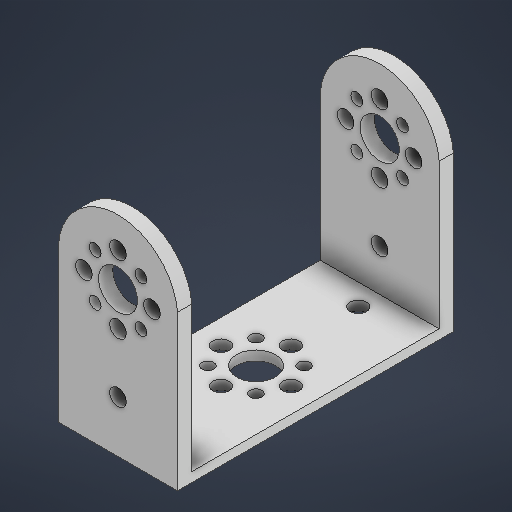
# Autodesk Inventor part: Medium FrameARRUMADO
Saved by Autodesk Inventor 2027 (Build 310192060, 192F)
## iProperties
Created: 2026-09-09
Part Number: Medium FrameARRUMADO
Material: Genérico
Document SubType Name: Modeling
Designer: joaop
Density: 1 g/cm^3
Appearance: Padrão
Author: joaop
Autodesk Inventor part; units mm, degrees
ref_plane "YZ Plane" through (0, 0, 0) normal (1, 0, 0) x (0, 1, 0)
ref_plane "XZ Plane" through (0, 0, 0) normal (0, 1, 0) x (-1, 0, 0)
ref_plane "XY Plane" through (0, 0, 0) normal (0, 0, 1) x (1, 0, 0)
sketch "Esboço1" plane through (0, 0, 0) normal (1, 0, 0) x (0, 1, 0)
  line L0 (0, 0) -> (50, 0)
  line L1 (50, 0) -> (50, 3)
  line L2 (50, 3) -> (2, 3)
  line L3 (2, 3) -> (2, 55)
  line L4 (2, 55) -> (50, 55)
  line L5 (50, 55) -> (50, 58)
  line L6 (50, 58) -> (0, 58)
  line L7 (0, 58) -> (0, 0)
  line L8 (2, 3) -> (0, 3)
  dimension "d84" = 52
  dimension "d85" = 3
  dimension "d86" = 3
  dimension "d87" = 3
  dimension "d90" = 2
  constraints: 18 end point, 3 point on line, 1 perpendicular
  measures "d84" distance between parallel lines of L2 L4
  measures "d85" distance of L4.end L5.end
  measures "d86" distance of L0.end L1.end
  measures "d87" distance from line of L2 L0.start
  measures "d90" distance between parallel lines of L7 L3
extrude "Extrusão1" add sketch "Esboço1" along normal blind 25
sketch "Esboço2" plane through (0, 0, 58) normal (0, 0, 1) x (1, 0, 0)
  line L0 (0, 0) -> (25, 0) projected
  circle A0 centre (12.5, 10.8) radius 1.75
  circle A1 centre (12.5, 30.4) radius 4.1
  circle A2 centre (12.5, 23.25) radius 1.75
  line L1 (12.5, 30.4) -> (16.5, 30.4) construction
  line L2 (12.5, 30.4) -> (19.3, 30.4) construction
  circle A3 centre (7.6917, 25.5917) radius 1.25
  circle A4 centre (19.65, 30.4) radius 1.75
  circle A5 centre (12.5, 37.55) radius 1.75
  circle A6 centre (5.35, 30.4) radius 1.75
  circle A7 centre (17.3083, 25.5917) radius 1.25
  circle A8 centre (17.3083, 35.2083) radius 1.25
  circle A9 centre (7.6917, 35.2083) radius 1.25
  line L3 (0, 0) -> (25, 0) projected
  line L4 (29.4538, 30.4) -> (-4.4538, 30.4)
  line L5 (12.5, 39.3) -> (12.5, 0)
  line L6 (12.5, 39.3) -> (12.5, 44)
  line L7 (25, 2) -> (25, 50) projected
  line L8 (25, 50) -> (25, 30.4)
  arc A10 (25, 30.4) -> (0, 30.4) centre (12.5, 31.4555) ccw
  line L9 (0, 2) -> (0, 50) projected
  line L10 (0, 50) -> (25, 50) projected
  line L11 (0, 32.511) -> (0, 50)
  line L12 (0, 50) -> (25, 50)
  line L13 (25, 50) -> (25, 32.511)
  line L14 (0, 32.511) -> (0, 30.4)
  line L15 (25, 32.511) -> (25, 30.4)
  line L16 (25, 32.511) -> (25, 50)
  point P0 (25, 32.511)
  dimension "d11" = 3.5
  dimension "d14" = 8.2
  dimension "d26" = 3.5
  dimension "d42" = 2.5
  dimension "d50" = 1.3
  dimension "d53" = 360
  dimension "d59" = 360
  dimension "d61" = 10.8
  dimension "d62" = 39.3
  dimension "d63" = 4.7
  constraints: 24 end point, 10 centre point, 6 point on line, 5 point on circle, 3 collinear, 3 midpoint, 3 vertical, 2 horizontal, 1 perpendicular, 1 vertical alignment, 20 other
  measures "d11" diameter of A0
  measures "d14" diameter of A1
  measures "d26" diameter of A2
  measures "d42" diameter of A3
  measures "d61" distance of L5.end A0.centre
  measures "d62" distance of L5.start L5.end
  measures "d63" distance of L5.start L6.end
extrude "Extrusão2" cut sketch "Esboço2" against normal through all contours A0 L5 | A1 L4 L5 | L5 L4 A1 | A2 L5 | L5 A2 | L5 A0 | A1 L5 L4 | L4 L5 A1 | L4 A6 | A6 L4 | L4 A4 | A4 L4 | L5 A5 | A5 L5 | A10 L9 L10 L7 | A3 | A7 | A8 | A9
sketch "Esboço4" plane through (0, 0, 0) normal (0, -1, 0) x (1, 0, 0)
  line L0 (0, 58) -> (25, 58) projected
  line L1 (14.25, 0) -> (10.75, 0) projected
  line L2 (25, 3) -> (25, 55) projected
  line L3 (0, 3) -> (0, 55) projected
  circle A0 centre (12.4993, 29.0025) radius 4.1
  circle A1 centre (12.4993, 21.6525) radius 1.75
  line L4 (12.4993, 29.0025) -> (16.4993, 29.0025) construction
  line L5 (12.4993, 29.0025) -> (19.2993, 29.0025) construction
  circle A2 centre (7.4434, 23.9467) radius 1.25
  circle A3 centre (19.8493, 29.0025) radius 1.75
  circle A4 centre (12.4993, 36.3525) radius 1.75
  circle A5 centre (5.1493, 29.0025) radius 1.75
  circle A6 centre (17.5551, 23.9467) radius 1.25
  circle A7 centre (17.5551, 34.0583) radius 1.25
  circle A8 centre (7.4434, 34.0583) radius 1.25
  circle A9 centre (12.5, 50.5) radius 1.75
  circle A10 centre (12.5, 7.5) radius 1.75
  line L6 (0, 0) -> (25, 0) projected
  line L7 (25, 58) -> (25, 0)
  line L8 (17.9, 3) -> (17.9, 0) projected
  line L9 (25, 58) -> (25, 0) projected
  line L10 (25, 29) -> (0, 29)
  line L11 (0, 58) -> (0, 0) projected
  line L12 (25, 58) -> (0, 58)
  line L13 (12.5, 58) -> (12.5, 0)
  point P0 (24.9565, 28.0304)
  dimension "d68" = 8.2
  dimension "d72" = 360
  dimension "d74" = 360
  dimension "d77" = 3.5
  dimension "d92" = 7.5
  dimension "d96" = 7.5
  dimension "d98" = 1.5
  dimension "d100" = 1.8
  dimension "d101" = 3.5
  dimension "d102" = 2.5
  dimension "d103" = 3.5
  constraints: 12 end point, 11 centre point, 4 midpoint, 3 horizontal, 1 parallel, 18 other
  measures "d68" diameter of A0
  measures "d77" diameter of A9
  measures "d92" distance from line of L6 A10.centre
  measures "d96" distance from line of L0 A9.centre
  measures "d101" diameter of A5
  measures "d102" diameter of A8
  measures "d103" diameter of A10
extrude "Extrusão3" cut sketch "Esboço4" against normal through all contours L13 A9 | A9 L13 | L10 A5 | A5 L10 | L13 A4 | A4 L13 | L10 A3 | A3 L10 | L10 L13 A0 | A0 L13 L10 | A0 L10 L13 | L13 L10 A0 | L13 A10 | A10 L13 | L13 A1 | A1 L13 | A2 | A6 | A7 | A8
